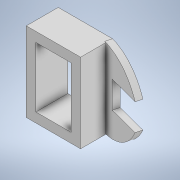
# Autodesk Inventor part: Servo front rightleft holder
Saved by Autodesk Inventor 2021 (Build 250183000, 183)
## iProperties
Created: 2021-02-11
Part Number: Servo front rightleft holder
Material: Generic
Document SubType Name: Modeling
Designer: chris
Density: 1 g/cm^3
Appearance: Default
Author: chris
Autodesk Inventor part; units mm, degrees
ref_plane "YZ Plane" through (0, 0, 0) normal (1, 0, 0) x (0, 1, 0)
ref_plane "XZ Plane" through (0, 0, 0) normal (0, 1, 0) x (-1, 0, 0)
sketch "Sketch1" plane through (0, 0, 0) normal (0, 0, 1) x (1, 0, 0)
  line L0 (-8.25, -14.15) -> (8.25, -14.15)
  line L1 (8.25, -14.15) -> (8.25, 14.15)
  line L2 (8.25, 14.15) -> (-8.25, 14.15)
  line L3 (-8.25, 14.15) -> (-8.25, -14.15)
  line L4 (-8.25, -14.15) -> (8.25, 14.15) construction
  line L5 (8.25, -14.15) -> (-8.25, 14.15) construction
  line L6 (-12.75, -18.65) -> (12.75, -18.65)
  line L7 (12.75, -18.65) -> (12.75, 18.65)
  line L8 (12.75, 18.65) -> (-12.75, 18.65)
  line L9 (-12.75, 18.65) -> (-12.75, -18.65)
  point P0 (0, 0)
  dimension "d0" = 16.5
  dimension "d1" = 28.3
  dimension "d2" = 4.5
  constraints: 20 end point, 4 parallel, 2 midpoint, 2 perpendicular, 1 horizontal, 3 other
  measures "d0" distance of L2.end L1.end
  measures "d1" distance of L1.end L0.end
  measures "d2" distance between parallel lines of L3 L9
extrude "Extrusion1" add sketch "Sketch1" along normal blind 15
ref_plane "Work Plane1" through (12.75, -18.65, 0) normal (-0.2534, 0, 0.9674) x (0, 1, 0)
sketch "Sketch2" plane through (12.75, -18.65, 0) normal (-0.2534, 0, 0.9674) x (0, 1, 0)
  line L0 (37.3, 0) -> (37.3, 24.6676) construction
  line L1 (37.3, 0) -> (0, 0)
  line L2 (0, 0) -> (0, -20)
  line L3 (0, -20) -> (37.3, -20)
  line L4 (37.3, -20) -> (37.3, 0)
  point P0 (18.65, 12.3338)
  dimension "d6" = 20
  constraints: 8 end point, 2 parallel, 2 vertical, 1 horizontal, 1 perpendicular
  measures "d6" distance of L2.end L1.end
extrude "Extrusion2" add sketch "Sketch2" along normal blind 3
sketch "Sketch5" plane through (12.75, -18.65, 0) normal (0.2534, 0, -0.9674) x (-0.9674, 0, -0.2534)
  line L0 (-35, 24.95) -> (-5, 24.95)
  line L1 (-5, 24.95) -> (-5, 12.35)
  line L2 (-5, 12.35) -> (-35, 12.35)
  line L3 (-35, 12.35) -> (-35, 24.95)
  line L4 (-20, 0) -> (-20, 37.3) construction
  line L5 (-35, 24.95) -> (-5, 12.35) construction
  line L6 (-5, 24.95) -> (-35, 12.35) construction
  point P0 (12.3338, 18.65)
  point P1 (-20, 18.65)
  dimension "d15" = 30
  dimension "d16" = 12.6
  constraints: 12 end point, 3 midpoint, 2 parallel, 1 horizontal, 1 perpendicular
  measures "d15" distance of L1.end L2.end
  measures "d16" distance of L0.end L1.end
extrude "Extrusion5" cut sketch "Sketch5" against normal blind 3
sketch "Sketch6" plane through (12.75, -18.65, 0) normal (0.2534, 0, -0.9674) x (-0.9674, 0, -0.2534)
  line L0 (0, 0) -> (-20, 0) construction
  line L1 (-20, 37.3) -> (0, 37.3) construction
  line L2 (-5, 24.95) -> (-20, 24.95) construction
  line L3 (-20, 12.35) -> (-5, 12.35) construction
  arc A0 (-20, 12.35) -> (0, 0) centre (0, 22.3693) ccw
  line L4 (-20, 0) -> (0, 0)
  line L5 (-20, 37.3) -> (-20, 24.95)
  line L6 (-20, 12.35) -> (-20, 0)
  arc A1 (0, 37.3) -> (-20, 24.95) centre (0, 14.9307) ccw
  line L7 (-20, 37.3) -> (-0.7859, 37.3) construction
  line L8 (0, 37.3) -> (-20, 37.3)
  point P0 (12.3338, 18.65)
  point P1 (0, 0)
  constraints: 8 end point, 4 point on circle, 2 centre point, 2 tangent, 1 collinear
extrude "Extrusion6" cut sketch "Sketch6" against normal blind 3
body "Solid1"
